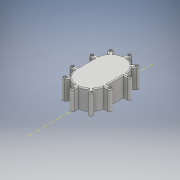
# Autodesk Inventor part: Gehaeuse_V1
Saved by Autodesk Inventor 2017 (Build 210142000, 142)
## iProperties
Created: 2019-05-23
Part Number: Gehaeuse_V1
Material: Generic
Document SubType Name: Modeling
Designer: Ole Simmering
Density: 1 g/cm^3
Appearance: Default
Author: Ole Simmering
Autodesk Inventor part; units mm, degrees
ref_plane "YZ Plane" through (0, 0, 0) normal (1, 0, 0) x (0, 1, 0)
ref_plane "XZ Plane" through (0, 0, 0) normal (0, 1, 0) x (-1, 0, 0)
ref_plane "XY Plane" through (0, 0, 0) normal (0, 0, 1) x (1, 0, 0)
sketch "Sketch1" plane through (0, 0, 0) normal (0, 0, 1) x (1, 0, 0)
  line L0 (0, 21.4588) -> (0, -11.275) construction
  line L1 (-75, 0) -> (-75, 50)
  arc A0 (0, 125) -> (-75, 50) centre (0, 50) ccw
  line L2 (-23.7356, 0) -> (21, 0) construction
  line L3 (75, 0) -> (75, 50)
  arc A1 (75, 50) -> (0, 125) centre (0, 50) ccw
  line L4 (-75, 0) -> (-75, -50)
  arc A2 (-75, -50) -> (0, -125) centre (0, -50) ccw
  arc A3 (0, -125) -> (75, -50) centre (0, -50) ccw
  line L5 (75, 0) -> (75, -50)
  point P0 (0, 0)
  dimension "d0" = 150
  dimension "d1" = 50
  constraints: 12 end point, 8 point on circle, 7 symmetric about line, 5 point on line, 4 centre point, 2 vertical, 1 horizontal, 1 tangent, 3 other
  measures "d0" diameter of L1 L0
  measures "d1" distance of L1.start L1.end
extrude "Extrusion1" add sketch "Sketch1" along normal blind 100
shell "Shell1" thickness 10 removed faces 1 at (-25, -16.6667, 0)
sketch "Sketch2" plane through (0, 0, 0) normal (0, 0, -1) x (-1, 0, 0)
  arc A0 (75, 50) -> (-75, 50) centre (0, 50) ccw construction
  line L0 (-75, 50) -> (-75, -50) construction
  arc A1 (-75, -50) -> (75, -50) centre (0, -50) ccw construction
  line L1 (75, -50) -> (75, 50) construction
  line L2 (-120, 50) -> (125, 50) construction
  line L3 (-75, 40) -> (-95, 40)
  arc A2 (-105, 50) -> (-95, 40) centre (-95, 50) ccw
  line L4 (-75, 60) -> (-95, 60)
  arc A3 (-95, 60) -> (-105, 50) centre (-95, 50) ccw
  circle A4 centre (-95, 50) radius 4
  line L5 (-75, 40) -> (-71.3179, 40)
  line L6 (-71.3179, 40) -> (-71.3179, 60)
  line L7 (-71.3179, 60) -> (-75, 60)
  line L8 (-45.9619, 110.1041) -> (-60.1041, 124.2462)
  line L9 (-43.3583, 107.5004) -> (-45.9619, 110.1041)
  line L10 (-57.5004, 93.3583) -> (-43.3583, 107.5004)
  line L11 (-60.1041, 95.9619) -> (-57.5004, 93.3583)
  line L12 (-60.1041, 95.9619) -> (-74.2462, 110.1041)
  arc A5 (-74.2462, 124.2462) -> (-74.2462, 110.1041) centre (-67.1751, 117.1751) ccw
  arc A6 (-60.1041, 124.2462) -> (-74.2462, 124.2462) centre (-67.1751, 117.1751) ccw
  circle A7 centre (-67.1751, 117.1751) radius 4
  line L13 (10, 125) -> (10, 145)
  line L14 (10, 121.3179) -> (10, 125)
  line L15 (-10, 121.3179) -> (10, 121.3179)
  line L16 (-10, 125) -> (-10, 121.3179)
  line L17 (-10, 125) -> (-10, 145)
  arc A8 (0, 155) -> (-10, 145) centre (0, 145) ccw
  arc A9 (10, 145) -> (0, 155) centre (0, 145) ccw
  circle A10 centre (0, 145) radius 4
  line L18 (60.1041, 95.9619) -> (74.2462, 110.1041)
  line L19 (57.5004, 93.3583) -> (60.1041, 95.9619)
  line L20 (43.3583, 107.5004) -> (57.5004, 93.3583)
  line L21 (45.9619, 110.1041) -> (43.3583, 107.5004)
  line L22 (45.9619, 110.1041) -> (60.1041, 124.2462)
  arc A11 (74.2462, 124.2462) -> (60.1041, 124.2462) centre (67.1751, 117.1751) ccw
  arc A12 (74.2462, 110.1041) -> (74.2462, 124.2462) centre (67.1751, 117.1751) ccw
  circle A13 centre (67.1751, 117.1751) radius 4
  line L23 (75, 40) -> (95, 40)
  line L24 (71.3179, 40) -> (75, 40)
  line L25 (71.3179, 60) -> (71.3179, 40)
  line L26 (75, 60) -> (71.3179, 60)
  line L27 (75, 60) -> (95, 60)
  arc A14 (105, 50) -> (95, 60) centre (95, 50) ccw
  arc A15 (95, 40) -> (105, 50) centre (95, 50) ccw
  circle A16 centre (95, 50) radius 4
  line L28 (-156.066, 0) -> (206, 0) construction
  arc A17 (-75, -50) -> (75, -50) centre (0, -50) ccw construction
  line L29 (-120, -50) -> (125, -50) construction
  line L30 (-75, -40) -> (-95, -40)
  arc A18 (-95, -40) -> (-105, -50) centre (-95, -50) ccw
  arc A19 (-105, -50) -> (-95, -60) centre (-95, -50) ccw
  line L31 (-75, -60) -> (-95, -60)
  circle A20 centre (-95, -50) radius 4
  line L32 (-75, -40) -> (-71.3179, -40)
  line L33 (-71.3179, -40) -> (-71.3179, -60)
  line L34 (-71.3179, -60) -> (-75, -60)
  line L35 (-45.9619, -110.1041) -> (-60.1041, -124.2462)
  line L36 (-43.3583, -107.5004) -> (-45.9619, -110.1041)
  line L37 (-57.5004, -93.3583) -> (-43.3583, -107.5004)
  line L38 (-60.1041, -95.9619) -> (-57.5004, -93.3583)
  line L39 (-60.1041, -95.9619) -> (-74.2462, -110.1041)
  arc A21 (-74.2462, -110.1041) -> (-74.2462, -124.2462) centre (-67.1751, -117.1751) ccw
  arc A22 (-74.2462, -124.2462) -> (-60.1041, -124.2462) centre (-67.1751, -117.1751) ccw
  circle A23 centre (-67.1751, -117.1751) radius 4
  line L40 (10, -125) -> (10, -145)
  line L41 (10, -121.3179) -> (10, -125)
  line L42 (-10, -121.3179) -> (10, -121.3179)
  line L43 (-10, -125) -> (-10, -121.3179)
  line L44 (-10, -125) -> (-10, -145)
  arc A24 (-10, -145) -> (0, -155) centre (0, -145) ccw
  arc A25 (0, -155) -> (10, -145) centre (0, -145) ccw
  circle A26 centre (0, -145) radius 4
  line L45 (60.1041, -95.9619) -> (74.2462, -110.1041)
  line L46 (57.5004, -93.3583) -> (60.1041, -95.9619)
  line L47 (43.3583, -107.5004) -> (57.5004, -93.3583)
  line L48 (45.9619, -110.1041) -> (43.3583, -107.5004)
  line L49 (45.9619, -110.1041) -> (60.1041, -124.2462)
  arc A27 (60.1041, -124.2462) -> (74.2462, -124.2462) centre (67.1751, -117.1751) ccw
  arc A28 (74.2462, -124.2462) -> (74.2462, -110.1041) centre (67.1751, -117.1751) ccw
  circle A29 centre (67.1751, -117.1751) radius 4
  line L50 (75, -40) -> (95, -40)
  line L51 (71.3179, -40) -> (75, -40)
  line L52 (71.3179, -60) -> (71.3179, -40)
  line L53 (75, -60) -> (71.3179, -60)
  line L54 (75, -60) -> (95, -60)
  arc A30 (95, -60) -> (105, -50) centre (95, -50) ccw
  arc A31 (105, -50) -> (95, -40) centre (95, -50) ccw
  circle A32 centre (95, -50) radius 4
  point P0 (0, 0)
  dimension "d6" = 20
  dimension "d7" = 10
  dimension "d8" = 8
  dimension "d9" = 3.6821
  dimension "d12" = 180
  constraints: 106 end point, 50 symmetric about line, 42 point on circle, 31 centre point, 10 coincident, 8 point on line, 4 horizontal, 2 perpendicular, 1 tangent, 86 other
  measures "d6" distance of L3.start L3.end
  measures "d7" radius of A2
  measures "d8" diameter of A4
  measures "d9" distance of L3.start L5.end
extrude "Extrusion2" add sketch "Sketch2" against normal blind 100
fillet "Fillet1" radius 5 40 edges at (-10, 134.6652, 100) (10, 134.6652, 100) (0, 155, 100) (-74.2462, 124.2462, 100) (-66.9384, 102.7962, 100) (-52.7962, 116.9384, 100) (-105, 50, 100) (-84.6652, 60, 100) (-85, 40, 100) (-105, -50, 100) (-84.6652, -60, 100) (-85, -40, 100) (-74.2462, -124.2462, 100) (-52.7962, -116.9384, 100) (-66.9384, -102.7962, 100) (0, -155, 100) (10, -134.6652, 100) (-10, -134.6652, 100) (105, 50, 100) (85, 40, 100) (84.6652, 60, 100) (52.7962, 116.9384, 100) (66.9384, 102.7962, 100) (74.2462, 124.2462, 100) (105, -50, 100) (84.6652, -60, 100) (85, -40, 100) (74.2462, -124.2462, 100) (52.7962, -116.9384, 100) (66.9384, -102.7962, 100) (75, 0, 100) (69.291, 78.7013, 100) (28.7013, 119.291, 100) (-28.7013, 119.291, 100) (-69.291, 78.7013, 100) (-75, 0, 100) (-69.291, -78.7013, 100) (-28.7013, -119.291, 100) (28.7013, -119.291, 100) (69.291, -78.7013, 100)
sketch "Sketch3" plane through (0, 0, 100) normal (0, 0, 1) x (1, 0, 0)
  line L0 (5, 145) -> (5, 119.8212) projected
  circle A0 centre (0, 145) radius 4 projected
  line L1 (-5, 119.8212) -> (-5, 145) projected
  arc A1 (-5, 119.8212) -> (-45.8355, 102.9066) centre (0, 50) ccw projected
  line L2 (-63.6396, 120.7107) -> (-45.8355, 102.9066) projected
  circle A2 centre (-67.1751, 117.1751) radius 4 projected
  line L3 (-52.9066, 95.8355) -> (-70.7107, 113.6396) projected
  arc A3 (-52.9066, 95.8355) -> (-69.8212, 55) centre (0, 50) ccw projected
  line L4 (-95, 55) -> (-69.8212, 55) projected
  circle A4 centre (-95, 50) radius 4 projected
  line L5 (-70, 45) -> (-95, 45) projected
  line L6 (-70, -45) -> (-70, 45) projected
  line L7 (-95, -45) -> (-70, -45) projected
  circle A5 centre (-95, -50) radius 4 projected
  line L8 (-69.8212, -55) -> (-95, -55) projected
  arc A6 (-69.8212, -55) -> (-52.9066, -95.8355) centre (0, -50) ccw projected
  line L9 (-70.7107, -113.6396) -> (-52.9066, -95.8355) projected
  circle A7 centre (-67.1751, -117.1751) radius 4 projected
  line L10 (-45.8355, -102.9066) -> (-63.6396, -120.7107) projected
  arc A8 (-45.8355, -102.9066) -> (-5, -119.8212) centre (0, -50) ccw projected
  line L11 (-5, -145) -> (-5, -119.8212) projected
  circle A9 centre (0, -145) radius 4 projected
  line L12 (5, -119.8212) -> (5, -145) projected
  arc A10 (5, -119.8212) -> (45.8355, -102.9066) centre (0, -50) ccw projected
  line L13 (63.6396, -120.7107) -> (45.8355, -102.9066) projected
  circle A11 centre (67.1751, -117.1751) radius 4 projected
  line L14 (52.9066, -95.8355) -> (70.7107, -113.6396) projected
  arc A12 (52.9066, -95.8355) -> (69.8212, -55) centre (0, -50) ccw projected
  line L15 (95, -55) -> (69.8212, -55) projected
  circle A13 centre (95, -50) radius 4 projected
  line L16 (70, -45) -> (95, -45) projected
  line L17 (70, 45) -> (70, -45) projected
  line L18 (95, 45) -> (70, 45) projected
  circle A14 centre (95, 50) radius 4 projected
  line L19 (69.8212, 55) -> (95, 55) projected
  arc A15 (69.8212, 55) -> (52.9066, 95.8355) centre (0, 50) ccw projected
  line L20 (70.7107, 113.6396) -> (52.9066, 95.8355) projected
  circle A16 centre (67.1751, 117.1751) radius 4 projected
  line L21 (45.8355, 102.9066) -> (63.6396, 120.7107) projected
  arc A17 (45.8355, 102.9066) -> (5, 119.8212) centre (0, 50) ccw projected
  line L22 (-87.4944, 50) -> (-91.2472, 43.5)
  line L23 (-91.2472, 43.5) -> (-98.7528, 43.5)
  line L24 (-98.7528, 43.5) -> (-102.5056, 50)
  line L25 (-102.5056, 50) -> (-98.7528, 56.5)
  line L26 (-98.7528, 56.5) -> (-91.2472, 56.5)
  line L27 (-91.2472, 56.5) -> (-87.4944, 50)
  line L28 (-59.9253, 119.1177) -> (-61.8679, 111.8679)
  line L29 (-61.8679, 111.8679) -> (-69.1177, 109.9253)
  line L30 (-65.2326, 124.425) -> (-59.9253, 119.1177)
  line L31 (-69.1177, 109.9253) -> (-74.425, 115.2326)
  line L32 (-72.4824, 122.4824) -> (-65.2326, 124.425)
  line L33 (-74.425, 115.2326) -> (-72.4824, 122.4824)
  line L34 (6.5, 141.2472) -> (0, 137.4944)
  line L35 (0, 137.4944) -> (-6.5, 141.2472)
  line L36 (6.5, 148.7528) -> (6.5, 141.2472)
  line L37 (-6.5, 141.2472) -> (-6.5, 148.7528)
  line L38 (0, 152.5056) -> (6.5, 148.7528)
  line L39 (-6.5, 148.7528) -> (0, 152.5056)
  line L40 (69.1177, 109.9253) -> (61.8679, 111.8679)
  line L41 (61.8679, 111.8679) -> (59.9253, 119.1177)
  line L42 (74.425, 115.2326) -> (69.1177, 109.9253)
  line L43 (59.9253, 119.1177) -> (65.2326, 124.425)
  line L44 (72.4824, 122.4824) -> (74.425, 115.2326)
  line L45 (65.2326, 124.425) -> (72.4824, 122.4824)
  line L46 (91.2472, 43.5) -> (87.4944, 50)
  line L47 (87.4944, 50) -> (91.2472, 56.5)
  line L48 (98.7528, 43.5) -> (91.2472, 43.5)
  line L49 (91.2472, 56.5) -> (98.7528, 56.5)
  line L50 (102.5056, 50) -> (98.7528, 43.5)
  line L51 (98.7528, 56.5) -> (102.5056, 50)
  line L52 (-158, 0) -> (164.7563, 0) construction
  arc A18 (3, -142.3542) -> (-3, -142.3542) centre (0, -145) ccw
  arc A19 (-63.183, -117.4256) -> (-67.4256, -113.183) centre (-67.1751, -117.1751) ccw
  arc A20 (-92.3542, -53) -> (-92.3542, -47) centre (-95, -50) ccw
  arc A21 (92.3542, -47) -> (92.3542, -53) centre (95, -50) ccw
  arc A22 (67.4256, -113.183) -> (63.183, -117.4256) centre (67.1751, -117.1751) ccw
  line L53 (-87.4944, -50) -> (-91.2472, -43.5)
  line L54 (-91.2472, -43.5) -> (-98.7528, -43.5)
  line L55 (-98.7528, -43.5) -> (-102.5056, -50)
  line L56 (-102.5056, -50) -> (-98.7528, -56.5)
  line L57 (-98.7528, -56.5) -> (-91.2472, -56.5)
  line L58 (-91.2472, -56.5) -> (-87.4944, -50)
  line L59 (-59.9253, -119.1177) -> (-61.8679, -111.8679)
  line L60 (-61.8679, -111.8679) -> (-69.1177, -109.9253)
  line L61 (-65.2326, -124.425) -> (-59.9253, -119.1177)
  line L62 (-69.1177, -109.9253) -> (-74.425, -115.2326)
  line L63 (-72.4824, -122.4824) -> (-65.2326, -124.425)
  line L64 (-74.425, -115.2326) -> (-72.4824, -122.4824)
  line L65 (6.5, -141.2472) -> (0, -137.4944)
  line L66 (0, -137.4944) -> (-6.5, -141.2472)
  line L67 (6.5, -148.7528) -> (6.5, -141.2472)
  line L68 (-6.5, -141.2472) -> (-6.5, -148.7528)
  line L69 (0, -152.5056) -> (6.5, -148.7528)
  line L70 (-6.5, -148.7528) -> (0, -152.5056)
  line L71 (69.1177, -109.9253) -> (61.8679, -111.8679)
  line L72 (61.8679, -111.8679) -> (59.9253, -119.1177)
  line L73 (74.425, -115.2326) -> (69.1177, -109.9253)
  line L74 (59.9253, -119.1177) -> (65.2326, -124.425)
  line L75 (72.4824, -122.4824) -> (74.425, -115.2326)
  line L76 (65.2326, -124.425) -> (72.4824, -122.4824)
  line L77 (91.2472, -43.5) -> (87.4944, -50)
  line L78 (87.4944, -50) -> (91.2472, -56.5)
  line L79 (98.7528, -43.5) -> (91.2472, -43.5)
  line L80 (91.2472, -56.5) -> (98.7528, -56.5)
  line L81 (102.5056, -50) -> (98.7528, -43.5)
  line L82 (98.7528, -56.5) -> (102.5056, -50)
  arc A23 (63.6396, -120.7107) -> (70.7107, -113.6396) centre (67.1751, -117.1751) ccw projected
  arc A24 (95, -55) -> (95, -45) centre (95, -50) ccw projected
  arc A25 (95, 45) -> (95, 55) centre (95, 50) ccw projected
  arc A26 (70.7107, 113.6396) -> (63.6396, 120.7107) centre (67.1751, 117.1751) ccw projected
  arc A27 (5, 145) -> (-5, 145) centre (0, 145) ccw projected
  arc A28 (-63.6396, 120.7107) -> (-70.7107, 113.6396) centre (-67.1751, 117.1751) ccw projected
  arc A29 (-95, 55) -> (-95, 45) centre (-95, 50) ccw projected
  arc A30 (-95, -45) -> (-95, -55) centre (-95, -50) ccw projected
  arc A31 (-70.7107, -113.6396) -> (-63.6396, -120.7107) centre (-67.1751, -117.1751) ccw projected
  arc A32 (-5, -145) -> (5, -145) centre (0, -145) ccw projected
  point P0 (0, 0)
  point P1 (0, 145)
  point P2 (0, -50)
  point P3 (0, -50)
  point P4 (0, -50)
  point P5 (0, -145)
  dimension "d18" = 13
  dimension "d21" = 180
  constraints: 122 end point, 43 symmetric about line, 10 point on circle, 5 centre point, 2 coincident, 2 horizontal, 1 point on line, 71 other
  measures "d18" distance between parallel lines of L23 L26
extrude "Extrusion3" cut sketch "Sketch3" against normal blind 15 contours A27 L1 L35 L37 L39 L38 L36 L34 L0 | L0 L34 L35 L1 A27 | L41 L43 L45 L44 L42 L40 L20 A26 L21 | L21 A26 L20 L40 L41 | L28 L29 L3 A28 L2 | L2 A28 L3 L29 L31 L33 L32 L30 L28 | L47 L49 L51 L50 L48 L46 L18 A25 L19 | L19 A25 L18 L46 L47 | L27 L22 L5 A29 L4 | L4 A29 L5 L22 L23 L24 L25 L26 L27 | L77 L79 L81 L82 L80 L78 L15 A24 L16 | L16 A24 L15 L78 L77 | L53 L58 L8 A30 L7 | L7 A30 L8 L58 L57 L56 L55 L54 L53 | L71 L73 L75 L76 L74 L72 L13 A23 L14 | L14 A23 L13 L72 L71 | L60 L59 L10 A31 L9 | L9 A31 L10 L59 L61 L63 L64 L62 L60 | L65 L67 L69 L70 L68 L66 L11 A32 L12 | L12 A32 L11 L66 L65 | A0 | A2 | A4 | A5 | A7 | A9 | A11 | A13 | A14 | A16
sketch "Sketch4" plane through (0, 0, 0) normal (0, 0, -1) x (-1, 0, 0)
  line L0 (0, 265) -> (0, -376) construction
  constraints: 2 end point
body "Solid1"
